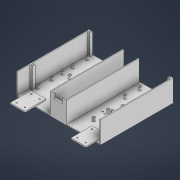
# Autodesk Inventor part: Grundplatte_hinten
Saved by Autodesk Inventor 2021 (Build 250183000, 183)
## iProperties
Created: 2021-01-26
Part Number: Grundplatte_hinten
Material: Generisch
Document SubType Name: Modeling
Designer: Ctroi
Density: 1 g/cm^3
Appearance: Vorgabe
Author: Ctroi
Autodesk Inventor part; units mm, degrees
ref_plane "YZ Plane" through (0, 0, 0) normal (1, 0, 0) x (0, 1, 0)
ref_plane "XZ Plane" through (0, 0, 0) normal (0, 1, 0) x (-1, 0, 0)
ref_plane "XY Plane" through (0, 0, 0) normal (0, 0, 1) x (1, 0, 0)
sketch "Skizze1" plane through (0, 0, 0) normal (0, 1, 0) x (-1, 0, 0)
  line L0 (-100, -87.5) -> (100, -87.5)
  line L1 (100, -87.5) -> (100, 87.5)
  line L2 (100, 87.5) -> (-100, 87.5)
  line L3 (-100, 87.5) -> (-100, -87.5)
  line L4 (0, -122.5) -> (0, 122.5) projected
  line L5 (-140, 0) -> (140, 0) projected
  point P0 (0, 0)
  dimension "d0" = 200
  dimension "d1" = 175
  constraints: 8 end point, 2 parallel, 1 horizontal, 1 perpendicular, 2 other
  measures "d0" distance of L1.end L2.end
  measures "d1" distance of L0.end L1.end
extrude "Extrusion1" add sketch "Skizze1" along normal blind 2
sketch "Skizze2" plane through (0, 2, 0) normal (0, 1, 0) x (1, 0, 0)
  line L0 (-90, -112.5) -> (-55, -112.5)
  line L1 (-55, -112.5) -> (-55, -62.5)
  line L2 (-55, -62.5) -> (-90, -62.5)
  line L3 (-90, -62.5) -> (-90, -112.5)
  line L4 (-100, -87.5) -> (100, -87.5) projected
  line L5 (-100, 87.5) -> (-100, -87.5) projected
  line L6 (0, 127.5) -> (0, -152.5) projected
  line L7 (90, -112.5) -> (55, -112.5)
  line L8 (55, -112.5) -> (55, -62.5)
  line L9 (55, -62.5) -> (90, -62.5)
  line L10 (90, -62.5) -> (90, -112.5)
  point P0 (0, 0)
  dimension "d4" = 35
  dimension "d5" = 50
  dimension "d6" = 10
  constraints: 16 end point, 4 symmetric about line, 2 parallel, 1 horizontal, 1 perpendicular, 1 other
  measures "d4" distance of L2.end L1.end
  measures "d5" distance of L1.end L0.end
  measures "d6" distance between parallel lines of L5 L3
extrude "Extrusion2" add sketch "Skizze2" along normal blind 3
sketch "Skizze3" plane through (0, 5, 0) normal (0, 1, 0) x (1, 0, 0)
  circle A0 centre (-82.5, -105) radius 1.6
  circle A1 centre (-62.5, -105) radius 1.6
  circle A2 centre (-82.5, -70) radius 1.6
  circle A3 centre (-62.5, -70) radius 1.6
  line L0 (-55, -112.5) -> (-55, -62.5) projected
  line L1 (-90, -62.5) -> (-90, -112.5) projected
  line L2 (-90, -112.5) -> (-55, -112.5) projected
  line L3 (-55, -62.5) -> (-90, -62.5) projected
  line L4 (0, 127.5) -> (0, -152.5) projected
  circle A4 centre (82.5, -105) radius 1.6
  circle A5 centre (62.5, -105) radius 1.6
  circle A6 centre (82.5, -70) radius 1.6
  circle A7 centre (62.5, -70) radius 1.6
  point P0 (0, 0)
  dimension "d9" = 3.2
  dimension "d10" = 3.2
  dimension "d11" = 3.2
  dimension "d12" = 3.2
  dimension "d13" = 7.5
  dimension "d14" = 7.5
  dimension "d15" = 7.5
  dimension "d16" = 7.5
  dimension "d17" = 7.5
  dimension "d18" = 7.5
  dimension "d19" = 7.5
  dimension "d20" = 7.5
  constraints: 8 centre point, 4 symmetric about line, 4 other
  measures "d9" diameter of A0
  measures "d10" diameter of A1
  measures "d11" diameter of A2
  measures "d12" diameter of A3
  measures "d13" distance from line of L0 A3.centre
  measures "d14" distance from line of L1 A2.centre
  measures "d15" distance from line of L1 A0.centre
  measures "d16" distance from line of L0 A1.centre
  measures "d17" distance from line of L2 A1.centre
  measures "d18" distance from line of L2 A0.centre
  measures "d19" distance from line of L3 A2.centre
  measures "d20" distance from line of L3 A3.centre
extrude "Extrusion3" cut sketch "Skizze3" against normal up to surface (5 mm away) contours A0 | A1 | A2 | A3 | A4 | A5 | A6 | A7
sketch "Skizze4" plane through (0, 2, 0) normal (0, 1, 0) x (1, 0, 0)
  line L0 (100, 87.5) -> (-100, 87.5) projected
  line L1 (0, 122.5) -> (0, -122.5) projected
  line L2 (-55, -87.5) -> (55, -87.5) projected
  line L3 (-100, 87.5) -> (-100, -87.5) projected
  line L4 (-17.5, 85.5) -> (-17.5, 85.5)
  line L5 (90, -87.5) -> (100, -87.5) projected
  line L6 (100, -87.5) -> (98, -87.5)
  line L7 (98, -87.5) -> (98, 85.5)
  line L8 (98, 85.5) -> (100, 85.5)
  line L9 (100, 85.5) -> (100, -87.5)
  line L10 (-100, -87.5) -> (-90, -87.5) projected
  line L11 (-100, -87.5) -> (-98, -87.5)
  line L12 (-98, -87.5) -> (-98, 85.5)
  line L13 (-98, 85.5) -> (-100, 85.5)
  line L14 (-100, 85.5) -> (-100, -87.5)
  line L15 (98, 85.5) -> (92, 85.5)
  line L16 (92, 85.5) -> (92, 79.5)
  line L17 (92, 79.5) -> (98, 79.5)
  line L18 (98, 79.5) -> (98, 85.5)
  line L19 (-98, 85.5) -> (-92, 85.5)
  line L20 (-92, 85.5) -> (-92, 79.5)
  line L21 (-92, 79.5) -> (-98, 79.5)
  line L22 (-98, 79.5) -> (-98, 85.5)
  line L23 (92, -57.5) -> (92, -51.5)
  line L24 (92, -51.5) -> (98, -51.5)
  line L25 (98, -51.5) -> (98, -87.5)
  line L26 (-92, -57.5) -> (-92, -51.5)
  line L27 (-92, -51.5) -> (-98, -51.5)
  line L28 (-98, -51.5) -> (-98, -87.5)
  line L29 (92, -57.5) -> (98, -57.5)
  line L30 (-98, -57.5) -> (-92, -57.5)
  line L31 (-19.5, -87.5) -> (19.5, -87.5)
  line L32 (19.5, -87.5) -> (19.5, 85.5)
  line L33 (20.25, 87.5) -> (-18.75, 87.5)
  line L34 (-19.5, 85.5) -> (-19.5, -87.5)
  line L35 (-17.5, -85.5) -> (17.5, -85.5)
  line L36 (17.5, -85.5) -> (17.5, 85.5)
  line L37 (-17.5, 85.5) -> (-17.5, -85.5)
  line L38 (-17.5, 85.5) -> (-19.5, 85.5)
  line L39 (17.5, 85.5) -> (19.5, 85.5)
  point P0 (-100, 85.5)
  point P1 (-98, 79.5)
  point P2 (98, 79.5)
  point P3 (-98, -51.5)
  point P4 (-92, -62.5)
  point P5 (98, -51.5)
  point P6 (92, -62.5)
  point P7 (98, -51.5)
  point P8 (-98, -51.5)
  point P9 (19.5, -87.5)
  dimension "d38" = 2
  dimension "d39" = 2
  dimension "d41" = 2
  dimension "d42" = 6
  dimension "d43" = 6
  dimension "d44" = 6
  dimension "d45" = 6
  dimension "d66" = 6
  dimension "d68" = 6
  dimension "d121" = 6
  dimension "d122" = 30
  dimension "d123" = 6
  dimension "d124" = 30
  dimension "d125" = 90
  dimension "d127" = 8
  dimension "d128" = 8
  dimension "d129" = 98
  dimension "d130" = 114
  dimension "d132" = 150
  dimension "d134" = 150
  dimension "d149" = 150
  dimension "d151" = 8
  dimension "d152" = 98
  dimension "d153" = 114
  dimension "d154" = 98
  dimension "d155" = 150
  dimension "d157" = 2
  dimension "d158" = 100
  dimension "d172" = 2
  dimension "d173" = 2
  dimension "d174" = 17.5
  dimension "d175" = 17.5
  dimension "d176" = 2
  dimension "d177" = 2
  constraints: 68 end point, 13 parallel, 9 perpendicular, 5 horizontal, 5 point on line, 1 other
  measures "d38" distance of L7.end L8.end
  measures "d39" distance of L13.end L12.end
  measures "d41" distance between parallel lines of L0 L8
  measures "d42" distance of L17.end L16.end
  measures "d43" distance of L16.end L15.end
  measures "d44" distance of L20.end L21.end
  measures "d45" distance of L19.end L20.end
  measures "d66" distance of L23.end L24.end
  measures "d68" distance of L27.end L26.end
  measures "d121" distance between parallel lines of L24 L29
  measures "d122" distance between parallel lines of L5 L29
  measures "d123" distance between parallel lines of L27 L30
  measures "d124" distance between parallel lines of L10 L30
  measures "d125" angle of L25 L0
  measures "d127" distance between parallel lines of L0 L21
  measures "d128" distance from line of point (98, 79.5) L0
  measures "d129" distance from line of point (98, 79.5) L1
  measures "d134" distance from line of point (92, -62.5) L0
  measures "d149" distance from line of point (-92, -62.5) L0
  measures "d151" distance from line of point (-98, 79.5) L0
  measures "d152" distance from line of point (-98, 79.5) L1
  measures "d154" distance from line of point (-98, -51.5) L1
  measures "d157" distance from line of point (-100, 85.5) L0
  measures "d158" distance from line of point (-100, 85.5) L1
  measures "d172" distance between parallel lines of L34 L37
  measures "d173" distance between parallel lines of L2 L35
  measures "d174" distance between parallel lines of L1 L37
  measures "d175" distance between parallel lines of L1 L36
  measures "d176" distance from line of L0 L4.end
  measures "d177" distance between parallel lines of L0 L39
extrude "Extrusion7" add sketch "Skizze4" along normal blind 50
sketch "Skizze7" plane through (100, 2, -85.5) normal (0, 0, -1) x (-1, 0, 0)
  circle A0 centre (4, 40) radius 2
  circle A1 centre (4, 10) radius 2
  line L0 (0, 0) -> (200, 0) projected
  line L1 (8, 0) -> (8, 50) projected
  line L2 (0, 50) -> (8, 50) projected
  circle A2 centre (196, 10) radius 2
  line L3 (192, 0) -> (192, 50) projected
  circle A3 centre (196, 40) radius 2
  line L4 (192, 50) -> (200, 50) projected
  point P0 (100, -2)
  dimension "d82" = 4
  dimension "d83" = 4
  dimension "d84" = 10
  dimension "d85" = 4
  dimension "d86" = 4
  dimension "d87" = 10
  dimension "d88" = 4
  dimension "d89" = 4
  dimension "d90" = 10
  dimension "d91" = 4
  dimension "d92" = 10
  dimension "d93" = 4
  constraints: 4 centre point
  measures "d82" diameter of A0
  measures "d83" diameter of A1
  measures "d84" distance from line of L0 A1.centre
  measures "d85" distance from line of L1 A1.centre
  measures "d86" distance from line of L1 A0.centre
  measures "d87" distance from line of L2 A0.centre
  measures "d88" diameter of A2
  measures "d89" distance from line of L3 A2.centre
  measures "d90" distance from line of L0 A2.centre
  measures "d91" diameter of A3
  measures "d92" distance from line of L4 A3.centre
  measures "d93" distance from line of L3 A3.centre
extrude "Extrusion8" cut sketch "Skizze7" against normal up to surface (6 mm away)
sketch "Skizze8" plane through (0, 52, 0) normal (0, 1, 0) x (1, 0, 0)
  circle A0 centre (95, 82.5) radius 2
  line L0 (100, 85.5) -> (92, 85.5) projected
  line L1 (92, 85.5) -> (92, 79.5) projected
  circle A1 centre (-95, 82.5) radius 2
  line L2 (-92, 85.5) -> (-100, 85.5) projected
  line L3 (-92, 79.5) -> (-92, 85.5) projected
  circle A2 centre (-95, -54.5) radius 2
  line L4 (-92, -51.5) -> (-98, -51.5) projected
  line L5 (-92, -57.5) -> (-92, -51.5) projected
  circle A3 centre (95, -54.5) radius 2
  line L6 (98, -51.5) -> (92, -51.5) projected
  line L7 (92, -51.5) -> (92, -57.5) projected
  point P0 (0, 0)
  point P1 (-92, -75)
  point P2 (92, -75)
  dimension "d96" = 4
  dimension "d97" = 3
  dimension "d98" = 3
  dimension "d99" = 4
  dimension "d100" = 3
  dimension "d101" = 3
  dimension "d102" = 4
  dimension "d103" = 3
  dimension "d104" = 3
  dimension "d105" = 4
  dimension "d106" = 3
  dimension "d107" = 3
  constraints: 4 centre point
  measures "d96" diameter of A0
  measures "d97" distance from line of L0 A0.centre
  measures "d98" distance from line of L1 A0.centre
  measures "d99" diameter of A1
  measures "d100" distance from line of L2 A1.centre
  measures "d101" distance from line of L3 A1.centre
  measures "d102" diameter of A2
  measures "d103" distance from line of L4 A2.centre
  measures "d104" distance from line of L5 A2.centre
  measures "d105" diameter of A3
  measures "d106" distance from line of L6 A3.centre
  measures "d107" distance from line of L7 A3.centre
extrude "Extrusion9" cut sketch "Skizze8" against normal blind 5
sketch "Skizze9" plane through (0, 2, 0) normal (0, 1, 0) x (1, 0, 0)
  circle A0 centre (-10, -69.5) radius 1.6
  line L0 (-55, -87.5) -> (-90, -87.5) projected
  line L1 (0, 122.5) -> (0, -122.5) projected
  circle A1 centre (10, -69.5) radius 1.6
  circle A2 centre (-42.961, -20.609) radius 1.6
  circle A3 centre (-35.444, -17.873) radius 1.6
  circle A4 centre (42.961, -20.609) radius 1.6
  circle A5 centre (35.444, -17.873) radius 1.6
  point P0 (0, 0)
  point P1 (0, -87.5)
  dimension "d110" = 3.2
  dimension "d111" = 18
  dimension "d112" = 10
  dimension "d115" = 3.2
  dimension "d116" = 3.2
  dimension "d117" = 66.891
  dimension "d118" = 69.627
  dimension "d119" = 42.961
  dimension "d120" = 35.444
  constraints: 6 centre point, 3 symmetric about line, 3 other
  measures "d110" diameter of A0
  measures "d111" distance from line of L0 A0.centre
  measures "d112" distance from line of L1 A0.centre
  measures "d115" diameter of A2
  measures "d116" diameter of A3
  measures "d117" distance from line of L0 A2.centre
  measures "d118" distance from line of L0 A3.centre
  measures "d119" distance from line of L1 A2.centre
  measures "d120" distance from line of L1 A3.centre
extrude "Extrusion10" cut sketch "Skizze9" against normal up to surface (2 mm away)
sketch "Skizze10" plane through (17.5, 2, 85.5) normal (0, 0, -1) x (-1, 0, 0)
  line L0 (37, 50) -> (-2, 50) projected
  line L1 (7.5, 50) -> (27.5, 50)
  line L2 (27.5, 50) -> (27.5, 40)
  line L3 (27.5, 40) -> (7.5, 40)
  line L4 (7.5, 40) -> (7.5, 50)
  line L5 (0, 0) -> (0, 50) projected
  point P0 (17.5, -2)
  dimension "d178" = 20
  dimension "d179" = 10
  dimension "d180" = 7.5
  constraints: 8 end point, 2 parallel, 1 horizontal, 1 perpendicular, 1 point on line
  measures "d178" distance of L2.end L3.end
  measures "d179" distance of L1.end L2.end
  measures "d180" distance between parallel lines of L5 L4
extrude "Extrusion11" cut sketch "Skizze10" against normal up to surface (2 mm away)
fillet "Rundung1" radius 2 1 edges at (0, 42, 87.5)
sketch "Skizze11" plane through (0, 2, 0) normal (0, 1, 0) x (1, 0, 0)
  circle A0 centre (-90, -47.5) radius 3.5
  circle A1 centre (-44, -47.5) radius 3.5
  circle A2 centre (-90, -13.5) radius 3.5
  circle A3 centre (-44, -13.5) radius 3.5
  line L0 (-98, -51.5) -> (-98, 79.5) projected
  line L1 (-55, -62.5) -> (-90, -62.5) projected
  line L2 (0, 127.5) -> (0, -152.5) projected
  circle A4 centre (90, -47.5) radius 3.5
  circle A5 centre (44, -47.5) radius 3.5
  circle A6 centre (90, -13.5) radius 3.5
  circle A7 centre (44, -13.5) radius 3.5
  circle A8 centre (-90, 36.5) radius 3.5
  circle A9 centre (-90, 71) radius 3.5
  circle A10 centre (-35, 36.5) radius 3.5
  circle A11 centre (-35, 71) radius 3.5
  circle A12 centre (90, 36.5) radius 3.5
  circle A13 centre (90, 71) radius 3.5
  circle A14 centre (35, 36.5) radius 3.5
  circle A15 centre (35, 71) radius 3.5
  circle A16 centre (-90, 11.5) radius 3.5
  circle A17 centre (-72, 11.5) radius 3.5
  circle A18 centre (-54, 11.5) radius 3.5
  circle A19 centre (90, 11.5) radius 3.5
  circle A20 centre (72, 11.5) radius 3.5
  circle A21 centre (54, 11.5) radius 3.5
  point P0 (0, 0)
  dimension "d184" = 7
  dimension "d185" = 7
  dimension "d186" = 7
  dimension "d187" = 7
  dimension "d188" = 8
  dimension "d189" = 15
  dimension "d190" = 15
  dimension "d191" = 46
  dimension "d192" = 8
  dimension "d193" = 46
  dimension "d194" = 34
  dimension "d195" = 34
  dimension "d196" = 7
  dimension "d197" = 7
  dimension "d198" = 7
  dimension "d199" = 7
  dimension "d200" = 8
  dimension "d201" = 8
  dimension "d202" = 50
  dimension "d203" = 34.5
  dimension "d204" = 55
  dimension "d205" = 50
  dimension "d206" = 55
  dimension "d207" = 34.5
  dimension "d241" = 7
  dimension "d242" = 7
  dimension "d243" = 7
  dimension "d244" = 25
  dimension "d245" = 8
  dimension "d246" = 25
  dimension "d247" = 25
  dimension "d248" = 18
  dimension "d249" = 18
  constraints: 22 centre point, 11 symmetric about line, 11 other
  measures "d184" diameter of A0
  measures "d185" diameter of A1
  measures "d186" diameter of A2
  measures "d187" diameter of A3
  measures "d188" distance from line of L0 A0.centre
  measures "d189" distance from line of L1 A0.centre
  measures "d190" distance from line of L1 A1.centre
  measures "d191" distance of A0.centre A1.centre
  measures "d192" distance from line of L0 A2.centre
  measures "d193" distance of A2.centre A3.centre
  measures "d194" distance of A0.centre A2.centre
  measures "d195" distance of A1.centre A3.centre
  measures "d196" diameter of A8
  measures "d197" diameter of A9
  measures "d198" diameter of A10
  measures "d199" diameter of A11
  measures "d200" distance from line of L0 A8.centre
  measures "d201" distance from line of L0 A9.centre
  measures "d202" distance of A2.centre A8.centre
  measures "d203" distance of A8.centre A9.centre
  measures "d204" distance of A8.centre A10.centre
  measures "d205" vertical distance of A3.centre A10.centre
  measures "d206" distance of A9.centre A11.centre
  measures "d207" distance of A10.centre A11.centre
  measures "d241" diameter of A16
  measures "d242" diameter of A17
  measures "d243" diameter of A18
  measures "d244" distance of A2.centre A16.centre
  measures "d245" distance from line of L0 A16.centre
  measures "d246" vertical distance of A2.centre A17.centre
  measures "d247" vertical distance of A2.centre A18.centre
  measures "d248" distance of A16.centre A17.centre
  measures "d249" distance of A17.centre A18.centre
extrude "Extrusion12" add sketch "Skizze11" along normal blind 7
sketch "Skizze12" plane through (-35, 9, -71) normal (0, 1, 0) x (1, 0, 0)
  circle A0 centre (-55, -118.5) radius 2
  circle A1 centre (-55, -118.5) radius 3.5 projected
  circle A2 centre (-55, -118.5) radius 3.5
  circle A3 centre (-55, -84.5) radius 3.5 projected
  circle A4 centre (-55, -84.5) radius 2
  circle A5 centre (-55, -84.5) radius 3.5
  circle A6 centre (-55, -34.5) radius 2
  circle A7 centre (-55, -34.5) radius 3.5 projected
  circle A8 centre (-55, -34.5) radius 3.5
  circle A9 centre (-55, 0) radius 3.5 projected
  circle A10 centre (0, 0) radius 3.5 projected
  circle A11 centre (0, -34.5) radius 3.5 projected
  circle A12 centre (-9, -84.5) radius 3.5 projected
  circle A13 centre (-9, -118.5) radius 3.5 projected
  circle A14 centre (-55, 0) radius 3.5
  circle A15 centre (-55, 0) radius 2
  circle A16 centre (0, 0) radius 3.5 projected
  circle A17 centre (0, 0) radius 2
  circle A18 centre (0, -34.5) radius 2
  circle A19 centre (-9, -84.5) radius 2
  circle A20 centre (-9, -118.5) radius 2
  circle A21 centre (79, -118.5) radius 3.5 projected
  circle A22 centre (79, -84.5) radius 3.5 projected
  circle A23 centre (70, -34.5) radius 3.5 projected
  circle A24 centre (70, 0) radius 3.5 projected
  circle A25 centre (125, 0) radius 3.5 projected
  circle A26 centre (125, -34.5) radius 3.5 projected
  circle A27 centre (125, -84.5) radius 3.5 projected
  circle A28 centre (125, -118.5) radius 3.5 projected
  circle A29 centre (79, -118.5) radius 2
  circle A30 centre (79, -84.5) radius 3.5 projected
  circle A31 centre (79, -84.5) radius 2
  circle A32 centre (70, -34.5) radius 3.5 projected
  circle A33 centre (70, -34.5) radius 2
  circle A34 centre (70, 0) radius 2
  circle A35 centre (125, -118.5) radius 3.5 projected
  circle A36 centre (125, -118.5) radius 2
  circle A37 centre (125, -84.5) radius 3.5 projected
  circle A38 centre (125, -84.5) radius 2
  circle A39 centre (125, -34.5) radius 3.5 projected
  circle A40 centre (125, -34.5) radius 2
  circle A41 centre (125, 0) radius 2
  circle A42 centre (-55, -59.5) radius 3.5 projected
  circle A43 centre (-37, -59.5) radius 3.5 projected
  circle A44 centre (-19, -59.5) radius 3.5 projected
  circle A45 centre (89, -59.5) radius 3.5 projected
  circle A46 centre (107, -59.5) radius 3.5 projected
  circle A47 centre (125, -59.5) radius 3.5 projected
  circle A48 centre (-55, -59.5) radius 2
  circle A49 centre (-37, -59.5) radius 2
  circle A50 centre (-19, -59.5) radius 2
  circle A51 centre (89, -59.5) radius 2
  circle A52 centre (107, -59.5) radius 2
  circle A53 centre (125, -59.5) radius 2
  point P0 (35, -71)
  dimension "d210" = 4
  dimension "d211" = 0
  dimension "d212" = 0
  dimension "d213" = 7
  dimension "d216" = 4
  dimension "d217" = 1.5
  dimension "d218" = 4
  dimension "d219" = 0
  dimension "d220" = 0
  dimension "d221" = 1.5
  dimension "d225" = 7
  dimension "d226" = 4
  dimension "d227" = 4
  dimension "d228" = 4
  dimension "d229" = 4
  dimension "d230" = 4
  dimension "d231" = 4
  dimension "d232" = 4
  dimension "d233" = 4
  dimension "d234" = 4
  dimension "d235" = 4
  dimension "d236" = 4
  dimension "d237" = 4
  dimension "d238" = 4
  dimension "d250" = 4
  dimension "d251" = 4
  dimension "d252" = 4
  dimension "d253" = 4
  dimension "d254" = 4
  dimension "d255" = 4
  constraints: 26 centre point, 22 coincident
  measures "d210" diameter of A0
  measures "d211" distance of A1.centre A0.centre
  measures "d212" distance of A1.centre A0.centre
  measures "d213" diameter of A2
  measures "d216" diameter of A4
  measures "d217" radial gap between concentric circles of A4 A5
  measures "d218" diameter of A6
  measures "d219" distance of A7.centre A6.centre
  measures "d220" distance of A7.centre A6.centre
  measures "d221" radial gap between concentric circles of A6 A8
  measures "d225" diameter of A14
  measures "d226" diameter of A15
  measures "d227" diameter of A17
  measures "d228" diameter of A18
  measures "d229" diameter of A19
  measures "d230" diameter of A20
  measures "d231" diameter of A29
  measures "d232" diameter of A31
  measures "d233" diameter of A33
  measures "d234" diameter of A34
  measures "d235" diameter of A36
  measures "d236" diameter of A38
  measures "d237" diameter of A40
  measures "d238" diameter of A41
  measures "d250" diameter of A48
  measures "d251" diameter of A49
  measures "d252" diameter of A50
  measures "d253" diameter of A51
  measures "d254" diameter of A52
  measures "d255" diameter of A53
extrude "Extrusion13" cut sketch "Skizze12" against normal blind 8 contours A0 | A4 | A6 | A15 | A17 | A18 | A19 | A20 | A29 | A31 | A33 | A34 | A36 | A38 | A40 | A41 | A48 | A49 | A50 | A51 | A52 | A53
